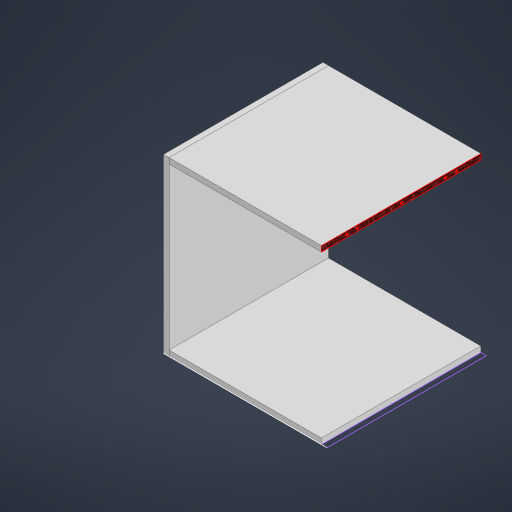
# Autodesk Inventor part: Деталь1
Saved by Autodesk Inventor 2023.4 (Build 274418000, 418)
## iProperties
Created: 2026-09-26
Part Number: Деталь1
Material: Типовые
Document SubType Name: Modeling
Designer: desig
Density: 1 g/cm^3
Appearance: По умолчанию
Author: desig
Autodesk Inventor part; units mm, degrees
ref_plane "YZ Plane" through (0, 0, 0) normal (1, 0, 0) x (0, 1, 0)
ref_plane "XZ Plane" through (0, 0, 0) normal (0, 1, 0) x (-1, 0, 0)
ref_plane "XY Plane" through (0, 0, 0) normal (0, 0, 1) x (1, 0, 0)
sketch "Эскиз1" plane through (0, 0, 0) normal (0, 1, 0) x (-1, 0, 0)
  line L0 (0, 0) -> (-16, 0)
  line L1 (-16, 0) -> (-16, -462.9097)
  line L2 (-16, -462.9097) -> (0, -462.9097)
  line L3 (0, -462.9097) -> (0, 0)
  line L4 (-458.1608, 0) -> (-474.1608, 0)
  line L5 (-474.1608, 0) -> (-474.1608, -462.9097)
  line L6 (-474.1608, -462.9097) -> (-458.1608, -462.9097)
  line L7 (-458.1608, -462.9097) -> (-458.1608, 0)
  line L8 (-16, -462.9097) -> (-458.1608, -462.9097)
  line L9 (-16, 0) -> (-458.1608, 0)
  dimension "d0" = 16
  dimension "d1" = 16
  dimension "d46" = 462.91
  dimension "d47" = 474.161
  constraints: 20 end point, 4 parallel, 3 horizontal, 3 perpendicular, 2 point on line
  measures "d0" distance of L1.end L2.end
  measures "d1" distance of L5.end L6.end
  measures "d46" distance of L2.end L0.start
  measures "d47" distance between parallel lines of L5 L3
extrude "Выдавливание1" add sketch "Эскиз1" along normal blind 500 contours L3 L2 L1 L0
extrude "Выдавливание2" add sketch "Эскиз1" against normal blind 16 from surface at 500 separate body contours L1 L8 L7 L9
extrude "Выдавливание3" add sketch "Эскиз1" along normal blind 16 separate body contours L1 L8 L7 L9
extrude "Выдавливание4" add sketch "Эскиз1" along normal up to surface (500 mm away) separate body contours L7 L6 L5 L4
sketch "DrillingSketch_1" plane through (458.1608, 484, -462.9097) normal (1, 0, 0) x (0, 0, -1)
  line L0 (0, 0) -> (-462.9097, 0) projected
  line L1 (0, 0) -> (0, 16) projected
  line L2 (0, 16) -> (-462.9097, 16) projected
  line L3 (-462.9097, 0) -> (-462.9097, 16) projected
  line L4 (0, 8) -> (-462.9097, 8) construction
  line L5 (-231.4549, 8) -> (-231.4549, -12) construction
  point P0 (-71.4549, 8)
  point P1 (-391.4549, 8)
  point P2 (-103.4549, 8)
  point P3 (-359.4549, 8)
  dimension "Шкант_глубина_в_пласть" = 10
  dimension "Минимальный_отступ_присадки_от_кромки_Каркас" = 70
  dimension "Long_edge_1" = 462.9097
  dimension "Расстояние_между_точками" = 320
  dimension "d1822" = 32
  constraints: 5 point on line, 4 end point, 4 midpoint, 2 symmetric about line, 1 perpendicular
  measures "Long_edge_1" distance of L4.start L4.end
  measures "Расстояние_между_точками" distance of point (-391.455, 8) point (-71.455, 8)
  measures "d1822" distance of point (-71.455, 8) point (-103.455, 8)
equation "\"d0\" = Толщина_каркаса"
equation "\"d1\" = Толщина_каркаса"
equation "\"d5\" = Толщина_каркаса"
equation "\"d7\" = Толщина_каркаса"
equation "\"Шкант_глубина_в_пласть\" = 10"
equation "\"Минимальный_отступ_присадки_от_кромки_Каркас\" = 70"
equation "\"Толщина_каркаса\" = 16"
equation "\"Стяжка_D\" = 15"
equation "\"Стяжка_h\" = 12.5"
equation "\"Стяжка_D_резьбыШтока\" = 5"
equation "\"Стяжка_D_телаШтока\" = 8"
equation "\"Стяжка_резьбыШтока_Петля_h\" = 12.5"
equation "\"Стяжка_отступ\" = 34"
equation "\"Конфирмат_D_вПласть\" = 8"
equation "\"Конфирмат_D_вТорец\" = 5"
equation "\"Толщина_каркаса_ящика\" = 16"
equation "\"Шкант_D\" = 8"
equation "\"Полкодержатель_D\" = 5"
equation "\"Полкодержатель_смещение_от_низа_полки\" = 5"
equation "\"Петля_D_присадки\" = 35"
equation "\"M_Конфирмат_глубина_резьбы\" = 35"
equation "\"M_Конфирмат_D_вПласть\" = 5"
equation "\"M_Конфирмат_D_вТорец\" = 3"
equation "\"Толщина_задн_ст_Володя\" = 3"
equation "\"Толщина_дна_ящика_Володя\" = 6"
equation "\"Минимальное_расстояния_от_заднСт_ящика_до_заднСт\" = 25"
equation "\"Западание_кромки_полки_за_каркас\" = 5"
